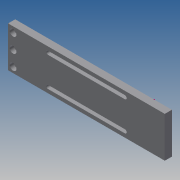
# Autodesk Inventor part: ASI_mesoSPIM_Bridge
Saved by Autodesk Inventor 2019 (Build 230136000, 136)
## iProperties
Created: 2020-05-15
Part Number: ASI_mesoSPIM_Bridge
Material: Generic
Document SubType Name: Modeling
Designer: voigt
Density: 1 g/cm^3
Appearance: Default
Author: voigt
Autodesk Inventor part; units mm, degrees
ref_plane "YZ Plane" through (0, 0, 0) normal (1, 0, 0) x (0, 1, 0)
ref_plane "XZ Plane" through (0, 0, 0) normal (0, 1, 0) x (-1, 0, 0)
ref_plane "XY Plane" through (0, 0, 0) normal (0, 0, 1) x (1, 0, 0)
sketch "Sketch1" plane through (0, 0, 0) normal (0, 0, 1) x (1, 0, 0)
  line L0 (-206.4864, -0.0159) -> (-206.4864, -68.5959) construction
  line L1 (-206.4864, -0.0159) -> (-222.6154, -0.0159) construction
  line L2 (-222.6154, -0.0159) -> (-222.6154, -68.5959) construction
  line L3 (-206.4864, -68.5959) -> (-222.6154, -68.5959) construction
  circle A0 centre (-214.5636, -21.8091) radius 3.3735 construction
  circle A1 centre (-214.5636, -46.8027) radius 3.3735 construction
  circle A2 centre (-214.5636, -9.3123) radius 2.5 construction
  circle A3 centre (-214.5636, -34.3059) radius 2.5 construction
  circle A4 centre (-214.5636, -59.2995) radius 2.5 construction
  line L4 (0.4039, -68.5877) -> (0.4039, -0.0077) construction
  line L5 (0.4039, -68.5877) -> (16.5329, -68.5877) construction
  line L6 (16.5329, -68.5877) -> (16.5329, -0.0077) construction
  line L7 (0.4039, -0.0077) -> (16.5329, -0.0077) construction
  circle A5 centre (8.4811, -46.7945) radius 3.3735 construction
  circle A6 centre (8.4811, -21.8009) radius 3.3735 construction
  circle A7 centre (8.4811, -59.2913) radius 2.5 construction
  circle A8 centre (8.4811, -34.2977) radius 2.5 construction
  circle A9 centre (8.4811, -9.3041) radius 2.5 construction
  line L8 (-223.0413, -0.0159) -> (16.9587, -0.0159)
  line L9 (16.9587, -0.0159) -> (16.9587, -68.5959)
  line L10 (16.9587, -68.5959) -> (-223.0413, -68.5959)
  line L11 (-223.0413, -68.5959) -> (-223.0413, -0.0159)
  line L12 (-103.0413, -534.726) -> (-103.0413, 430.7972) construction
  point P0 (0, 0)
  dimension "d0" = 240
  dimension "d23" = 120
  constraints: 10 end point, 3 parallel, 2 collinear, 1 horizontal, 1 perpendicular, 1 vertical, 2 other
  measures "d0" distance between parallel lines of L9 L11
  measures "d23" distance between parallel lines of L11 L12
extrude "Extrusion1" add sketch "Sketch1" along normal blind 12
sketch "Sketch3" plane through (0, 0, 0) normal (0, 0, -1) x (-1, 0, 0)
  circle A0 centre (65.542, -46.7868) radius 2.5 construction
  circle A1 centre (65.542, -21.7868) radius 2.5 construction
  circle A2 centre (165.542, -21.7868) radius 2.5 construction
  circle A3 centre (165.542, -46.7868) radius 2.5 construction
  circle A4 centre (140.542, -46.7868) radius 2.5 construction
  circle A5 centre (140.542, -21.7868) radius 2.5 construction
  circle A6 centre (65.542, -46.7868) radius 2.5 construction
  circle A7 centre (65.542, -21.7868) radius 2.5 construction
  circle A8 centre (40.542, -21.7868) radius 2.5 construction
  circle A9 centre (40.542, -46.7868) radius 2.5 construction
  point P0 (0, 0)
  constraints: 8 coincident
sketch "Sketch4" plane through (0, 0, 0) normal (0, 0, -1) x (-1, 0, 0)
  circle A0 centre (65.5413, -59.3059) radius 2.5 construction
  circle A1 centre (40.5413, -59.3059) radius 2.5 construction
  circle A2 centre (140.5413, -9.3059) radius 2.5 construction
  circle A3 centre (115.5413, -9.3059) radius 2.5 construction
  line L0 (40.5413, -59.3059) -> (172.5963, -59.3059) construction
  line L1 (167.5124, -9.3059) -> (3.0086, -9.3059) construction
  line L2 (223.0413, -0.0159) -> (-16.9587, -0.0159) construction
  line L3 (38.0413, -9.3059) -> (168.0413, -9.3059) construction
  line L4 (38.0413, -12.3559) -> (168.0413, -12.3559)
  line L5 (168.0413, -6.2559) -> (38.0413, -6.2559)
  arc A4 (38.0413, -6.2559) -> (38.0413, -12.3559) centre (38.0413, -9.3059) ccw
  arc A5 (168.0413, -12.3559) -> (168.0413, -6.2559) centre (168.0413, -9.3059) ccw
  line L6 (103.0413, 455.7975) -> (103.0413, -509.7257) construction
  line L7 (38.0413, -59.3059) -> (168.0413, -59.3059) construction
  line L8 (38.0413, -62.3559) -> (168.0413, -62.3559)
  line L9 (168.0413, -56.2559) -> (38.0413, -56.2559)
  arc A6 (38.0413, -56.2559) -> (38.0413, -62.3559) centre (38.0413, -59.3059) ccw
  arc A7 (168.0413, -62.3559) -> (168.0413, -56.2559) centre (168.0413, -59.3059) ccw
  point P0 (0, 0)
  point P1 (-16.9587, -0.0159)
  point P2 (103.0413, -9.3059)
  point P3 (103.0413, -59.3059)
  dimension "d10" = 9.29
  dimension "d11" = 6.1
  dimension "d12" = 65
  dimension "d13" = 65
  dimension "d14" = 6.1
  dimension "d15" = 65
  dimension "d16" = 65
  constraints: 22 end point, 8 point on circle, 8 tangent, 4 centre point, 3 point on line, 2 horizontal, 2 midpoint, 2 parallel, 1 horizontal alignment, 1 vertical, 4 other
  measures "d11" diameter of A5
  measures "d12" distance from line of L3.end L6
  measures "d13" distance from line of L6 L3.start
  measures "d14" diameter of A7
  measures "d15" distance from line of L6 L7.start
  measures "d16" distance from line of L6 L7.end
extrude "Extrusion2" cut sketch "Sketch4" against normal blind 12
sketch "Sketch5" plane through (0, 0, 0) normal (0, 0, -1) x (-1, 0, 0)
  line L0 (45.6373, -31.0674) -> (77.6413, -31.0674) construction
  arc A0 (168.0413, -12.3559) -> (168.0413, -6.2559) centre (168.0413, -9.3059) ccw construction
  arc A1 (168.0413, -62.3559) -> (168.0413, -56.2559) centre (168.0413, -59.3059) ccw construction
  arc A2 (38.0413, -6.2559) -> (38.0413, -12.3559) centre (38.0413, -9.3059) ccw construction
  arc A3 (38.0413, -56.2559) -> (38.0413, -62.3559) centre (38.0413, -59.3059) ccw construction
  line L1 (38.0413, -9.3059) -> (168.0413, -9.3059) construction
  line L2 (-16.9587, -0.0159) -> (223.0413, -0.0159) projected
  line L3 (38.0413, -14.5559) -> (168.0413, -14.5559)
  line L4 (168.0413, -4.0559) -> (38.0413, -4.0559)
  arc A4 (38.0413, -4.0559) -> (38.0413, -14.5559) centre (38.0413, -9.3059) ccw
  arc A5 (168.0413, -14.5559) -> (168.0413, -4.0559) centre (168.0413, -9.3059) ccw
  line L5 (38.0413, -59.3059) -> (168.0413, -59.3059) construction
  line L6 (38.0413, -64.5559) -> (168.0413, -64.5559)
  line L7 (168.0413, -54.0559) -> (38.0413, -54.0559)
  arc A6 (38.0413, -54.0559) -> (38.0413, -64.5559) centre (38.0413, -59.3059) ccw
  arc A7 (168.0413, -64.5559) -> (168.0413, -54.0559) centre (168.0413, -59.3059) ccw
  point P0 (0, 0)
  point P1 (103.0413, -9.3059)
  point P2 (103.0413, -59.3059)
  dimension "d19" = 10.5
  dimension "d20" = 10.5
  constraints: 16 end point, 8 point on circle, 8 tangent, 4 centre point, 3 parallel, 2 midpoint, 1 horizontal, 1 other
  measures "d19" diameter of A5
  measures "d20" diameter of A7
extrude "Extrusion3" cut sketch "Sketch5" against normal blind 6.5
sketch "Sketch6" plane through (0, 0, 12) normal (0, 0, 1) x (1, 0, 0)
  line L0 (0.4039, -68.5877) -> (0.4039, -0.0077) construction
  line L1 (0.4039, -68.5877) -> (16.5329, -68.5877) construction
  line L2 (16.5329, -68.5877) -> (16.5329, -0.0077) construction
  line L3 (0.4039, -0.0077) -> (16.5329, -0.0077) construction
  circle A0 centre (8.4811, -46.7945) radius 3.3735 construction
  circle A1 centre (8.4811, -21.8009) radius 3.3735 construction
  circle A2 centre (8.4811, -59.2913) radius 2.5 construction
  circle A3 centre (8.4811, -34.2977) radius 2.5 construction
  circle A4 centre (8.4811, -9.3041) radius 2.5 construction
  line L4 (-206.4864, -0.0159) -> (-206.4864, -68.5959) construction
  line L5 (-206.4864, -0.0159) -> (-222.6154, -0.0159) construction
  line L6 (-222.6154, -0.0159) -> (-222.6154, -68.5959) construction
  line L7 (-206.4864, -68.5959) -> (-222.6154, -68.5959) construction
  circle A5 centre (-214.5636, -21.8091) radius 3.3735 construction
  circle A6 centre (-214.5636, -46.8027) radius 3.3735 construction
  circle A7 centre (-214.5636, -9.3123) radius 2.5 construction
  circle A8 centre (-214.5636, -34.3059) radius 2.5 construction
  circle A9 centre (-214.5636, -59.2995) radius 2.5 construction
  point P0 (0, 0)
  constraints: 6 coincident
hole "Hole2" at (8.4811, -59.2913, 12) at (8.4811, -34.2977, 12) at (8.4811, -9.3041, 12) at (-214.5636, -59.2995, 12) at (-214.5636, -34.3059, 12) at (-214.5636, -9.3123, 12) direction (0, 0, -1) diameter 6.1 depth 20 tip angle 118 counterbore diameter 11.5 counterbore depth 7
body "Solid1"
